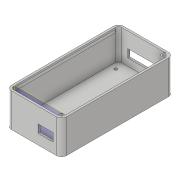
# Autodesk Inventor part: 00_Case_Powersupply_Galvo
Saved by Autodesk Inventor 2019.4 (Build 234330000, 330)
## iProperties
Created: 2021-10-06
Part Number: 00_Case_Powersupply_Galvo
Material: Generic
Document SubType Name: Modeling
Designer: diederichbenedict
Density: 1 g/cm^3
Appearance: Default
Author: diederichbenedict
Autodesk Inventor part; units mm, degrees
ref_plane "YZ Plane" through (0, 0, 0) normal (1, 0, 0) x (0, 1, 0)
ref_plane "XZ Plane" through (0, 0, 0) normal (0, 1, 0) x (-1, 0, 0)
ref_plane "XY Plane" through (0, 0, 0) normal (0, 0, 1) x (1, 0, 0)
sketch "Sketch1" plane through (0, 0, 0) normal (0, 1, 0) x (-1, 0, 0)
  line L0 (-19.5, -45) -> (19.5, -45) construction
  line L1 (19.5, -45) -> (19.5, 45) construction
  line L2 (19.5, 45) -> (-19.5, 45) construction
  line L3 (-19.5, 45) -> (-19.5, -45) construction
  line L4 (-19.5, -45) -> (19.5, 45) construction
  line L5 (19.5, -45) -> (-19.5, 45) construction
  line L6 (-27, -55) -> (27, -55)
  line L7 (27, -55) -> (27, 55)
  line L8 (27, 55) -> (-27, 55)
  line L9 (-27, 55) -> (-27, -55)
  line L10 (-27, -55) -> (27, 55) construction
  line L11 (27, -55) -> (-27, 55) construction
  circle A0 centre (19.5, 45) radius 1.45
  circle A1 centre (-19.5, 45) radius 1.45
  circle A2 centre (19.3553, -44.6662) radius 1.45
  circle A3 centre (-19.5, -45) radius 1.45
  point P0 (0, 0)
  dimension "d0" = 39
  dimension "d1" = 90
  dimension "d2" = 54
  dimension "d3" = 110
  dimension "d4" = 2.9
  dimension "d5" = 2.9
  dimension "d6" = 2.9
  dimension "d7" = 2.9
  constraints: 24 end point, 4 centre point, 4 midpoint, 4 parallel, 2 coincident, 2 horizontal, 2 perpendicular, 2 point on line
  measures "d0" distance of L2.end L1.end
  measures "d1" distance of L1.end L0.end
  measures "d2" distance of L8.end L7.end
  measures "d3" distance of L7.end L6.end
  measures "d4" diameter of A0
  measures "d5" diameter of A1
  measures "d6" diameter of A2
  measures "d7" diameter of A3
extrude "Extrusion1" add sketch "Sketch1" along normal blind 3
fillet "Fillet1" radius 5 4 edges at (27, 1.5, 55) (-27, 1.5, 55) (-27, 1.5, -55) (27, 1.5, -55)
sketch "Sketch2" plane through (0, 3, 0) normal (0, 1, 0) x (1, 0, 0)
  arc A0 (27, 50) -> (22, 55) centre (22, 50) ccw projected
  line L0 (22, 55) -> (-22, 55) projected
  arc A1 (-22, 55) -> (-27, 50) centre (-22, 50) ccw projected
  line L1 (-27, 50) -> (-27, -50) projected
  arc A2 (-27, -50) -> (-22, -55) centre (-22, -50) ccw projected
  line L2 (-22, -55) -> (22, -55) projected
  arc A3 (22, -55) -> (27, -50) centre (22, -50) ccw projected
  line L3 (27, -50) -> (27, 50) projected
  circle A4 centre (19.5, 45) radius 1.45 projected
  circle A5 centre (-19.3553, 44.6662) radius 1.45 projected
  circle A6 centre (19.5, -45) radius 1.45 projected
  circle A7 centre (-19.5, -45) radius 1.45 projected
  line L4 (-25, -50) -> (-25, 50)
  arc A8 (-22, 53) -> (-25, 50) centre (-22, 50) ccw
  line L5 (-22, 53) -> (22, 53)
  arc A9 (25, 50) -> (22, 53) centre (22, 50) ccw
  line L6 (25, 50) -> (25, -50)
  arc A10 (22, -53) -> (25, -50) centre (22, -50) ccw
  line L7 (22, -53) -> (-22, -53)
  arc A11 (-25, -50) -> (-22, -53) centre (-22, -50) ccw
  point P0 (0, 0)
  dimension "d11" = 2
  constraints: 8 end point, 8 point on circle, 4 centre point, 7 other
  measures "d11" distance between parallel lines of L1 L4
extrude "Extrusion2" add sketch "Sketch2" along normal blind 30 contours L3 A3 L2 A2 L1 A1 L0 A0
sketch "Sketch3" plane through (-22, 0, 55) normal (0, 0, 1) x (1, 0, 0)
  line L0 (41, 18) -> (26, 18)
  line L1 (26, 18) -> (26, 10)
  line L2 (26, 10) -> (41, 10)
  line L3 (41, 10) -> (41, 18)
  line L4 (41, 18) -> (26, 10) construction
  line L5 (26, 18) -> (41, 10) construction
  line L6 (49, 0) -> (49, 33) projected
  line L7 (0, 0) -> (44, 0) projected
  point P0 (22, 0)
  point P1 (33.5, 14)
  dimension "d14" = 8
  dimension "d15" = 10
  dimension "d16" = 15
  dimension "d17" = 8
  constraints: 12 end point, 2 midpoint, 2 parallel, 1 horizontal, 1 perpendicular
  measures "d14" distance between parallel lines of L3 L6
  measures "d15" distance between parallel lines of L7 L2
  measures "d16" distance between parallel lines of L3 L1
  measures "d17" distance between parallel lines of L0 L2
extrude "Extrusion3" cut sketch "Sketch3" against normal blind 30
sketch "Sketch4" plane through (22, 0, -55) normal (0, 0, -1) x (-1, 0, 0)
  line L0 (0, 0) -> (0, 33) projected
  line L1 (0, 0) -> (44, 0) projected
  line L2 (44, 33) -> (44, 0) projected
  line L3 (0, 33) -> (44, 33) projected
  line L4 (18, 10) -> (18, 18) construction
  line L5 (18, 18) -> (3, 18) construction
  line L6 (3, 18) -> (3, 10) construction
  line L7 (3, 10) -> (18, 10) construction
  line L8 (44, 0) -> (44, 33) construction
  line L9 (44, 0) -> (0, 0) construction
  line L10 (0, 33) -> (0, 0) construction
  line L11 (44, 33) -> (0, 33) construction
  line L12 (3, 10) -> (38, 10)
  line L13 (38, 10) -> (38, 18)
  line L14 (38, 18) -> (3, 18)
  line L15 (3, 18) -> (3, 10)
  point P0 (22, 0)
  dimension "d20" = 35
  constraints: 8 end point, 2 parallel, 1 horizontal, 1 perpendicular
  measures "d20" distance of L14.end L13.end
extrude "Extrusion4" cut sketch "Sketch4" against normal blind 30 contours L15 L14 L13 L12
sketch "Sketch5" plane through (0, 33, 0) normal (0, 1, 0) x (1, 0, 0)
  arc A0 (-25, -50) -> (-22, -53) centre (-22, -50) ccw projected
  arc A1 (22, -53) -> (25, -50) centre (22, -50) ccw projected
  arc A2 (25, 50) -> (22, 53) centre (22, 50) ccw projected
  arc A3 (-22, 53) -> (-25, 50) centre (-22, 50) ccw projected
  circle A4 centre (-23, -51) radius 1.45
  circle A5 centre (23, -51) radius 1.45
  circle A6 centre (-23, 51) radius 1.45
  arc A7 (-22, 53) -> (-25, 50) centre (-22, 50) ccw projected
  line L0 (-22, 53) -> (22, 53) projected
  arc A8 (25, 50) -> (22, 53) centre (22, 50) ccw projected
  line L1 (25, 50) -> (25, -50) projected
  arc A9 (22, -53) -> (25, -50) centre (22, -50) ccw projected
  line L2 (22, -53) -> (-22, -53) projected
  arc A10 (-25, -50) -> (-22, -53) centre (-22, -50) ccw projected
  line L3 (-25, -50) -> (-25, 50) projected
  arc A11 (27, 50) -> (22, 55) centre (22, 50) ccw projected
  line L4 (22, 55) -> (-22, 55) projected
  arc A12 (-22, 55) -> (-27, 50) centre (-22, 50) ccw projected
  line L5 (-27, 50) -> (-27, -50) projected
  arc A13 (-27, -50) -> (-22, -55) centre (-22, -50) ccw projected
  line L6 (-22, -55) -> (22, -55) projected
  arc A14 (22, -55) -> (27, -50) centre (22, -50) ccw projected
  line L7 (27, -50) -> (27, 50) projected
  arc A15 (-22, 51) -> (-23, 50) centre (-22, 50) ccw construction
  line L8 (-22, 51) -> (22, 51) construction
  arc A16 (23, 50) -> (22, 51) centre (22, 50) ccw construction
  line L9 (23, 50) -> (23, -50) construction
  arc A17 (22, -51) -> (23, -50) centre (22, -50) ccw construction
  line L10 (22, -51) -> (-22, -51) construction
  arc A18 (-23, -50) -> (-22, -51) centre (-22, -50) ccw construction
  line L11 (-23, -50) -> (-23, 50) construction
  line L12 (23, 51) -> (-23, 51) construction
  line L13 (-23, 51) -> (-23, -51) construction
  line L14 (-23, -51) -> (23, -51) construction
  line L15 (23, -51) -> (23, 51) construction
  line L16 (23, 51) -> (-23, -51) construction
  line L17 (-23, 51) -> (23, -51) construction
  line L18 (-25, 50) -> (-25, -50) projected
  arc A19 (-22, -53) -> (-25, -50) centre (-22.8913, -50.8913) ccw
  line L19 (-22, -53) -> (22, -53) projected
  arc A20 (25, -50) -> (22, -53) centre (22.921, -50.921) ccw
  arc A21 (-25, 50) -> (-22, 53) centre (-22.9063, 50.9063) ccw
  arc A22 (25, 50) -> (22, 53) centre (22, 50) ccw projected
  arc A23 (22, 53) -> (25, 50) centre (22.4561, 50.4561) ccw
  circle A24 centre (22.4561, 50.4561) radius 1.45
  circle A25 centre (-23, -51) radius 2.2361
  circle A26 centre (23, -51) radius 2.2361
  point P0 (0, 0)
  point P1 (24.1213, 52.1213)
  dimension "d23" = 2.9
  dimension "d24" = 2.9
  dimension "d25" = 2.9
  dimension "d27" = 2
  dimension "d28" = 2.9
  constraints: 20 end point, 17 point on circle, 12 centre point, 6 coincident, 4 point on line, 2 midpoint, 2 parallel, 1 horizontal, 1 perpendicular, 13 other
  measures "d23" diameter of A4
  measures "d24" diameter of A5
  measures "d25" diameter of A6
  measures "d27" distance between parallel lines of L3 L11
  measures "d28" diameter of A24
extrude "Extrusion5" add sketch "Sketch5" against normal blind 10 contours A26 A1 | A1 A26 | A2 A23
ref_plane "Work Plane1" through (22, 3, 50) normal (0, 0, -1) x (-1, 0, 0)
sketch "Sketch6" plane through (22, 3, 50) normal (0, 0, -1) x (-1, 0, 0)
  line L0 (46.829, 28.3524) -> (47.7477, 28.3524)
  line L1 (47.7477, 28.3524) -> (46.829, 24.7431)
  line L2 (46.829, 24.7431) -> (46.829, 28.3524)
  line L3 (22, 24.0878) -> (22, -17.3662)
  line L4 (-2.829, 28.3524) -> (-3.7477, 28.3524)
  line L5 (-3.7477, 28.3524) -> (-2.829, 24.7431)
  line L6 (-2.829, 24.7431) -> (-2.829, 28.3524)
  point P0 (22, -3)
  constraints: 14 end point, 3 symmetric about line, 1 horizontal, 1 perpendicular, 1 vertical
extrude "Extrusion6" cut sketch "Sketch6" along normal blind 100
body "Solid1"
